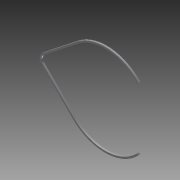
# Autodesk Inventor part: neck chain
Saved by Autodesk Inventor 2011 SP1 (Build 150282100, 282)
## iProperties
Created: 2012-01-20
Part Number: neck chain
Document SubType Name: Modeling
Designer: Christopher
Density: 1 g/cm^3
Author: Christopher
Autodesk Inventor part; units mm, degrees
ref_plane "YZ Plane" through (0, 0, 0) normal (1, 0, 0) x (0, 1, 0)
ref_plane "XZ Plane" through (0, 0, 0) normal (0, 1, 0) x (-1, 0, 0)
ref_plane "XY Plane" through (0, 0, 0) normal (0, 0, 1) x (1, 0, 0)
sketch "Sketch1" plane through (0, 0, 0) normal (0, 0, 1) x (1, 0, 0)
  line L0 (-11.8119, 27.5254) -> (114.7385, 127.5389)
  line L1 (-13.4704, -0.891) -> (100.5859, -114.9473)
  arc A0 (100.5859, -114.9473) -> (330.4805, -114.9473) centre (215.5332, 0) ccw
  arc A1 (330.4805, 114.9473) -> (114.7385, 127.5389) centre (215.5332, 0) ccw
  line L2 (-15.7492, 32.5074) -> (110.8012, 132.5209)
  arc A2 (339.3763, 114.8628) -> (110.8012, 132.5209) centre (215.5332, 0) ccw
  arc A3 (96.0958, -119.4374) -> (339.3763, -114.8628) centre (215.5332, 0) ccw
  line L3 (96.0958, -119.4374) -> (-17.9605, -5.3811)
  arc A4 (-15.7492, 32.5074) -> (-17.9605, -5.3811) centre (0, 12.5794) ccw
  arc A5 (-11.8119, 27.5254) -> (-13.4704, -0.891) centre (0, 12.5794) ccw
  line L4 (330.4805, 114.9473) -> (334.9706, 110.4572)
  line L5 (330.4805, -114.9473) -> (334.9706, -110.4572)
  line L6 (334.9706, -110.4572) -> (339.3763, -114.8628)
  line L7 (334.9706, 110.4572) -> (339.3763, 114.8628)
  point P0 (0, 0)
  dimension "d4" = 6.35
  dimension "d5" = 6.35
  constraints: 16 end point, 12 point on circle, 6 centre point, 2 coincident, 2 tangent, 2 other
  measures "d4" distance between parallel lines of L0 L2
  measures "d5" distance between parallel lines of L1 L3
extrude "Extrusion1" add sketch "Sketch1" against normal blind 6.35
body "Solid1"
